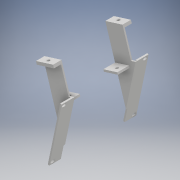
# Autodesk Inventor part: soportePantalla
Saved by Autodesk Inventor 2017 (Build 210142000, 142)
## iProperties
Part Number: soportePantalla
Material: Genérico
Document SubType Name: Modeling
Designer: Roberto
Density: 1 g/cm^3
Appearance: Valor por defecto
Author: Roberto
Autodesk Inventor part; units mm, degrees
ref_plane "Plano de trabajo1" through (0, 3.2, 0) normal (0, 1, 0) x (-1, 0, 0)
ref_plane "Plano de trabajo2" through (0, -3.2, 0) normal (0, 1, 0) x (-1, 0, 0)
sketch "Boceto3" plane through (0, 3.2, 0) normal (0, 1, 0) x (-1, 0, 0)
  line L0 (0, -6.196) -> (0, 0) projected
  line L1 (0, -6.196) -> (1.7583, -0.5473) projected
  line L2 (1.7583, -0.5473) -> (0, 0) projected
sketch "Boceto4" plane through (0, -3.2, 0) normal (0, 1, 0) x (-1, 0, 0)
  line L0 (0, -6.196) -> (0, 0) projected
  line L1 (0, -6.196) -> (1.7583, -0.5473) projected
  line L2 (1.7583, -0.5473) -> (0, 0) projected
extrude "Extrusión3" add sketch "Boceto4" along normal mid plane 0.15
extrude "Extrusión4" add sketch "Boceto3" along normal mid plane 0.15
ref_plane "Plano de trabajo3" through (0, -3.275, 0) normal (-0.2972, 0, 0.9548) x (0.9548, 0, 0.2972)
sketch "Boceto7" plane through (0, -3.275, 0) normal (-0.2972, 0, 0.9548) x (0.9548, 0, 0.2972)
  line L0 (-1.8415, 0.15) -> (0, 0.15) projected
  line L1 (-1.8415, 0) -> (-1.8415, 0.15) projected
  line L2 (0, 0) -> (-1.8415, 0) projected
  line L3 (-1.8415, 6.55) -> (0, 6.55) projected
  line L4 (-1.8415, 6.4) -> (-1.8415, 6.55) projected
  line L5 (0, 6.4) -> (-1.8415, 6.4) projected
  line L6 (0, 0.15) -> (0, 0) projected
  line L7 (0, 6.55) -> (0, 6.4) projected
  point P0 (0, 3.275)
extrude "Extrusión7" add sketch "Boceto7" along normal blind 2.92
sketch "Boceto8" plane through (0, 3.275, -6.196) normal (-0.9548, 0, -0.2972) x (-0.2972, 0, 0.9548)
  line L0 (0, -6.4) -> (8.836, -6.4) projected
  line L1 (0, -6.55) -> (8.836, -6.55) projected
  line L2 (0, 0) -> (8.836, 0) projected
  line L3 (0, -0.15) -> (8.836, -0.15) projected
  line L4 (8.836, -6.55) -> (8.836, -7.275)
  line L5 (8.836, -7.275) -> (8.536, -7.275)
  line L6 (8.536, -7.275) -> (8.536, -6.55)
  line L7 (5.916, -6.55) -> (8.836, -6.55) projected
  line L8 (8.836, -6.55) -> (8.536, -6.55)
  line L9 (8.916, -0.15) -> (8.916, 0) projected
  line L10 (8.836, 0) -> (8.836, 0.725)
  line L11 (8.836, 0.725) -> (8.536, 0.725)
  line L12 (8.536, 0.725) -> (8.536, 0)
  line L13 (8.536, 0) -> (8.836, 0)
  line L14 (0, -0.15) -> (0, 0) projected
  line L15 (0, -6.55) -> (0, -6.4) projected
  line L16 (8.836, 0) -> (8.836, -0.15) projected
  line L17 (8.836, -6.4) -> (8.836, -6.55) projected
  point P0 (5.916, -3.275)
  dimension "d19" = 0.725
  dimension "d20" = 0.3
  dimension "d21" = 0.725
  dimension "d22" = 0.3
  constraints: 16 end point, 4 perpendicular, 2 point on line, 2 vertical, 1 collinear
  measures "d19" distance of L4.start L4.end
  measures "d20" distance of L4.end L5.end
  measures "d21" distance of L9.end L10.end
  measures "d22" distance of L10.end L11.end
extrude "Extrusión8" add sketch "Boceto8" against normal blind 1.842 contours L4 L5 L6 L1 | L12 L11 L10 L2
sketch "Boceto9" plane through (-0.8678, -3.275, 2.7881) normal (-0.2972, 0, 0.9548) x (0.9548, 0, 0.2972)
  line L0 (0, 0.15) -> (-1.8415, 0.15) projected
  line L1 (-1.8415, 0.15) -> (-1.8415, -0.725) projected
  line L2 (-1.8415, -0.725) -> (0.0005, -0.725) projected
  line L3 (0.0005, 0) -> (0.0005, -0.725) projected
  line L4 (0, 0) -> (0.0005, 0) projected
  line L5 (0, 6.55) -> (0.0005, 6.55) projected
  line L6 (0.0005, 7.275) -> (0.0005, 6.55) projected
  line L7 (-1.8415, 7.275) -> (0.0005, 7.275) projected
  line L8 (-1.8415, 6.4) -> (-1.8415, 7.275) projected
  line L9 (-1.8415, 6.4) -> (0, 6.4) projected
  circle A0 centre (-0.9205, -0.325) radius 0.15
  circle A1 centre (-0.9205, 6.875) radius 0.15
  line L10 (0, 6.4) -> (0, 6.55) projected
  line L11 (0, 0) -> (0, 0.15) projected
  point P0 (0, 3.275)
  dimension "d27" = 0.3
  dimension "d28" = 0.3
  constraints: 2 centre point
  measures "d27" diameter of A0
  measures "d28" diameter of A1
extrude "Extrusión9" cut sketch "Boceto9" against normal blind 1.842 contours A0 | A1
ref_plane "Plano de trabajo5" through (0, 1.925, -0.8902) normal (0.2972, 0, -0.9548) x (-0.9548, 0, -0.2972)
sketch "Boceto12" plane through (0, 1.925, -0.8902) normal (0.2972, 0, -0.9548) x (-0.9548, 0, -0.2972)
  line L0 (3.1538, -5.05) -> (3.1538, -3.85) projected
  line L1 (1.5769, -3.85) -> (3.1538, -3.85) projected
  line L2 (1.5769, -5.05) -> (1.5769, -3.85) projected
  line L3 (1.5769, 1.2) -> (1.5769, 0) projected
  line L4 (3.1538, 0) -> (1.5769, 0) projected
  line L5 (3.1538, 1.2) -> (3.1538, 0) projected
  line L6 (1.5769, -3.85) -> (3.1538, -3.85) projected
  circle A0 centre (0.6559, -5.525) radius 0.15 projected
  circle A1 centre (0.6559, 0.525) radius 0.15
  circle A2 centre (0.6559, -4.375) radius 0.15
  line L7 (3.1538, 1.2) -> (1.5769, 1.2) projected
  line L8 (1.5769, -5.05) -> (3.1538, -5.05) projected
  point P0 (-0.2646, -1.925)
  dimension "d41" = 0.3
  dimension "d42" = 0.3
  constraints: 2 centre point
  measures "d41" diameter of A1
  measures "d42" diameter of A2
extrude "Extrusión12" cut sketch "Boceto12" against normal blind 1.2 contours A1 | A2
ref_plane "Plano de trabajo4" through (-0.1783, -3.125, -0.4137) normal (-0.2972, 0, 0.9548) x (0.9548, 0, 0.2972)
sketch "Boceto13" plane through (-0.1783, -3.125, -0.4137) normal (-0.2972, 0, 0.9548) x (0.9548, 0, 0.2972)
  circle A0 centre (0.6273, -0.475) radius 0.15 projected
  circle A1 centre (0.6273, 6.725) radius 0.15 projected
  line L0 (0.6273, 6.725) -> (0.6273, -0.475)
  circle A2 centre (0.6273, 0.675) radius 0.15
  circle A3 centre (0.6273, 5.575) radius 0.15
  point P0 (-0.2932, 3.125)
  dimension "d50" = 0.3
  dimension "d51" = 0.3
  constraints: 2 centre point, 2 end point, 2 point on line, 1 vertical
  measures "d50" diameter of A2
  measures "d51" diameter of A3
extrude "Extrusión13" cut sketch "Boceto13" against normal blind 10 contours A3 L0 | L0 A3 | A2 L0 | L0 A2
sketch "Boceto14" plane through (0, 3.275, 0) normal (0, 1, 0) x (1, 0, 0)
  line L0 (-2.537, -1.9543) -> (-2.6261, -2.2407) projected
  line L1 (-2.537, -1.9543) -> (-0.3978, -2.6202)
  line L2 (0, 0) -> (2.1391, -0.6659)
  line L3 (0, 0) -> (0, 6.196) projected
  line L4 (0, 0) -> (0.4774, -0.1486)
  line L5 (0, 0) -> (-0.2806, 5.2944)
  line L6 (0, 6.196) -> (-2.6261, -2.2407) projected
  line L7 (-0.2806, 5.2944) -> (0, 6.196)
  line L8 (0, 6.196) -> (0, 0)
  line L9 (0, 0) -> (-0.7787, -2.5016) projected
  line L10 (-0.2806, 5.2944) -> (0, 0)
  line L11 (0, 0) -> (-0.3893, 4.9452)
  line L12 (-0.3893, 4.9452) -> (0, 6.196)
  line L13 (-0.2806, 5.2944) -> (-0.3893, 4.9452)
  line L14 (0, 0) -> (-0.5085, 4.5623)
  line L15 (0, 6.196) -> (-2.537, -1.9543) projected
  line L16 (-0.3893, 4.9452) -> (-0.5085, 4.5623)
  point P0 (-1.5675, 1.1603)
  dimension "d54" = 0.5
  constraints: 24 end point, 4 point on line, 2 collinear, 1 perpendicular, 1 vertical
  measures "d54" distance of L3.start L4.end
extrude "Extrusión14" cut sketch "Boceto14" against normal blind 10 contours L6 L11 L14 | L5 L6 L3 | L11 L6 L5
sketch "Boceto15" plane through (0, 3.275, 0) normal (0, 1, 0) x (1, 0, 0)
  line L0 (-0.0139, -0.0029) -> (2.134, -0.6398)
  line L1 (0, 0) -> (0.4774, -0.1486)
  line L2 (0, 0) -> (-0.7787, -2.5016)
  line L3 (0.4774, -0.1486) -> (-0.0139, -0.0029)
  line L4 (0, 0) -> (-0.7787, -2.5016) projected
  line L5 (0, 0) -> (0.4774, -0.1486)
  line L6 (0, 0) -> (-0.5085, 4.5623) projected
  line L7 (-0.5085, 4.5623) -> (0, 0) projected
  line L8 (0.4774, -0.1486) -> (-0.5085, 4.5623)
  line L9 (-0.5085, 4.5623) -> (0, 0)
  line L10 (-0.0139, -0.0029) -> (0.4774, -0.1486)
  line L11 (0.4774, -0.1486) -> (-0.5085, 4.5623)
  line L12 (-0.539, 4.708) -> (-0.0139, -0.0029)
  dimension "d57" = 0.5
  constraints: 20 end point, 2 point on line, 1 collinear, 1 perpendicular
  measures "d57" distance of L1.start L1.end
extrude "Extrusión15" add sketch "Boceto15" against normal blind 0.15 contours L1 L6 L8
sketch "Boceto16" plane through (0, -3.275, 0) normal (0, -1, 0) x (1, 0, 0)
  line L0 (0, 0) -> (-0.8678, 2.7881) projected
  line L1 (-2.6261, 2.2407) -> (-0.8678, 2.7881) projected
  line L2 (-0.5085, -4.5623) -> (-2.6261, 2.2407) projected
  line L3 (-0.5085, -4.5623) -> (0.4774, 0.1486) projected
  line L4 (0.4774, 0.1486) -> (0, 0) projected
extrude "Extrusión16" add sketch "Boceto16" against normal blind 0.15
sketch "Boceto17" plane through (0, 3.125, 0) normal (0, -1, 0) x (1, 0, 0)
  line L0 (-2.6261, 2.2407) -> (-2.537, 1.9543) projected
  line L1 (-1.571, -1.1488) -> (-0.1388, -0.703)
  line L2 (-0.1388, -0.703) -> (-0.1983, -0.5121)
  line L3 (-0.1983, -0.5121) -> (-1.6305, -0.9579)
  line L4 (-1.6305, -0.9579) -> (-1.571, -1.1488)
  line L5 (-0.5085, -4.5623) -> (-2.537, 1.9543) projected
  line L6 (-1.571, -1.1488) -> (-0.1388, -0.703)
  line L7 (-0.1388, -0.703) -> (-0.1983, -0.5121)
  line L8 (-0.1983, -0.5121) -> (-1.6305, -0.9579)
  point P0 (0, 0)
  point P1 (-0.2806, -5.2944)
  point P2 (-0.3893, -4.9452)
  dimension "d62" = 3.55
  dimension "d63" = 1.5
  dimension "d64" = 0.2
  constraints: 14 end point, 5 perpendicular, 1 collinear
  measures "d62" distance of L0.start L1.start
  measures "d63" distance of L1.start L1.end
  measures "d64" distance of L1.end L2.end
extrude "Extrusión17" add sketch "Boceto17" along normal blind 1.2
sketch "Boceto18" plane through (0, -3.125, 0) normal (0, 1, 0) x (1, 0, 0)
  line L0 (-1.571, 1.1488) -> (-0.1388, 0.703) projected
  line L1 (-0.1388, 0.703) -> (-0.1983, 0.5121) projected
  line L2 (-0.1983, 0.5121) -> (-1.6305, 0.9579) projected
  line L3 (-1.6305, 0.9579) -> (-1.571, 1.1488) projected
  point P0 (0, 0)
extrude "Extrusión18" add sketch "Boceto18" along normal blind 1.2
sketch "Boceto19" plane through (-1.571, -3.125, -1.1488) normal (0.2972, 0, -0.9548) x (-0.9548, 0, -0.2972)
  circle A0 centre (-0.921, 6.725) radius 0.15 projected
  circle A1 centre (-0.921, -0.475) radius 0.15 projected
  circle A2 centre (-0.921, 5.575) radius 0.15
  circle A3 centre (-0.921, 0.675) radius 0.15
  point P0 (-1.8415, 3.125)
  dimension "d70" = 0.3
  dimension "d71" = 0.3
  constraints: 2 centre point
  measures "d70" diameter of A2
  measures "d71" diameter of A3
extrude "Extrusión19" cut sketch "Boceto19" against normal blind 1.2 contours A2 | A3
sketch "Boceto21" plane through (0.4774, 3.125, 0.1486) normal (0.9788, 0, -0.2048) x (-0.2048, 0, -0.9788)
  line L0 (0.2432, 0.15) -> (0, 0.15) projected
  arc A0 (6.096, -7.245) -> (5.796, -7.245) centre (5.946, -7.245) ccw
  line L1 (6.096, -7.245) -> (6.096, -7.345)
  arc A1 (5.796, -7.345) -> (6.096, -7.345) centre (5.946, -7.345) ccw
  line L2 (0, -7.595) -> (6.196, -7.595)
  line L3 (5.796, -7.345) -> (5.796, -7.245)
  arc A2 (0.4, -7.245) -> (0.1, -7.245) centre (0.25, -7.245) ccw
  line L4 (0.4, -7.245) -> (0.4, -7.345)
  arc A3 (0.1, -7.345) -> (0.4, -7.345) centre (0.25, -7.345) ccw
  line L5 (0.1, -7.345) -> (0.1, -7.245)
  line L6 (0.4, 1.095) -> (0.4, 0.995)
  line L7 (0.1, 0.995) -> (0.1, 1.095)
  arc A4 (0.4, 1.095) -> (0.1, 1.095) centre (0.25, 1.095) ccw
  arc A5 (5.796, 0.995) -> (6.096, 0.995) centre (5.946, 0.995) ccw
  line L8 (6.096, 1.095) -> (6.096, 0.995)
  arc A6 (6.096, 1.095) -> (5.796, 1.095) centre (5.946, 1.095) ccw
  line L9 (6.196, 1.345) -> (0, 1.345)
  arc A7 (0.1, 0.995) -> (0.4, 0.995) centre (0.25, 0.995) ccw
  line L10 (5.796, 0.995) -> (5.796, 1.095)
  line L11 (0, 0.15) -> (4.813, 0.15) projected
  line L12 (0, -6.4) -> (4.813, -6.4) projected
  line L13 (0, 0.15) -> (6.196, 0.15)
  line L14 (0, -6.4) -> (6.196, -6.4)
  line L15 (6.196, -7.595) -> (6.196, -6.4)
  line L16 (6.196, 0.15) -> (6.196, 1.345)
  line L17 (0, 1.345) -> (0, 0.15)
  line L18 (0, -6.4) -> (0, -7.595)
  point P0 (0, 1.345)
  constraints: 32 end point, 16 point on circle, 8 centre point, 2 perpendicular, 1 point on line
extrude "Extrusión21" add sketch "Boceto21" against normal blind 0.15
